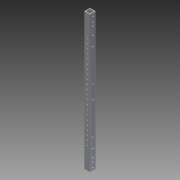
# Autodesk Inventor part: Chassis V1.500 Part1
Saved by Autodesk Inventor 2013 (Build 170138000, 138)
## iProperties
Created: 2013-01-05
Part Number: Chassis V1.500 Part1
Material: Aluminum 6061
Document SubType Name: Modeling
Designer: Moses
Density: 2.71 g/cm^3
Mass: 446.253 g
Surface Area: 1087.72 cm^2
Volume: 164.669 cm^3
Author: Moses
Autodesk Inventor part; units mm, degrees
ref_plane "YZ Plane" through (0, 0, 0) normal (1, 0, 0) x (0, 1, 0)
ref_plane "XZ Plane" through (0, 0, 0) normal (0, 1, 0) x (-1, 0, 0)
ref_plane "XY Plane" through (0, 0, 0) normal (0, 0, 1) x (1, 0, 0)
sketch "Sketch1" plane through (0, 0, 0) normal (0, 1, 0) x (-1, 0, 0)
  line L0 (0, 25.4) -> (25.4, 25.4)
  line L1 (25.4, 25.4) -> (25.4, 0)
  line L2 (25.4, 0) -> (0, 0)
  line L3 (0, 0) -> (0, 25.4)
  line L4 (22.225, 22.225) -> (3.175, 22.225)
  line L5 (3.175, 22.225) -> (3.175, 3.175)
  line L6 (3.175, 3.175) -> (22.225, 3.175)
  line L7 (22.225, 3.175) -> (22.225, 22.225)
  dimension "d0" = 25.4
  dimension "d1" = 25.4
  dimension "d2" = 3.175
  constraints: 16 end point, 4 parallel, 2 perpendicular, 1 coincident, 1 horizontal, 3 other
  measures "d0" distance of L1.end L2.end
  measures "d1" distance of L0.end L1.end
  measures "d2" distance between parallel lines of L0 L4
extrude "Extrusion1" add sketch "Sketch1" along normal blind 609.6
sketch "Sketch2" plane through (-25.4, 0, 25.4) normal (0, 0, 1) x (1, 0, 0)
  circle A0 centre (12.7, 491.5841) radius 3.302 projected
  circle A1 centre (12.7, 452.2611) radius 3.302 projected
  circle A2 centre (12.7, 412.9381) radius 3.302 projected
  circle A3 centre (12.7, 373.6152) radius 3.302 projected
  circle A4 centre (12.7, 334.2922) radius 3.302 projected
  circle A5 centre (12.7, 294.9693) radius 3.302 projected
  circle A6 centre (12.7, 255.6463) radius 3.302 projected
  circle A7 centre (12.7, 216.3233) radius 3.302 projected
  circle A8 centre (12.7, 177.0004) radius 3.302 projected
  circle A9 centre (12.7, 137.6774) radius 3.302 projected
  circle A10 centre (12.7, 98.3544) radius 3.302 projected
  circle A11 centre (12.7, 118.0159) radius 3.302 projected
  circle A12 centre (12.7, 157.3389) radius 3.302 projected
  circle A13 centre (12.7, 196.6619) radius 3.302 projected
  circle A14 centre (12.7, 235.9848) radius 3.302 projected
  circle A15 centre (12.7, 275.3078) radius 3.302 projected
  circle A16 centre (12.7, 314.6307) radius 3.302 projected
  circle A17 centre (12.7, 353.9537) radius 3.302 projected
  circle A18 centre (12.7, 393.2767) radius 3.302 projected
  circle A19 centre (12.7, 432.5996) radius 3.302 projected
  circle A20 centre (12.7, 471.9226) radius 3.302 projected
  circle A21 centre (12.7, 511.2456) radius 3.302 projected
  line L0 (0, 25.4) -> (25.4, 25.4) projected
  line L1 (0, 25.4) -> (0, 584.2) projected
  line L2 (25.4, 584.2) -> (0, 584.2) projected
  line L3 (25.4, 25.4) -> (25.4, 584.2) projected
extrude "Extrusion2" cut sketch "Sketch2" against normal through all contours A0 | A1 | A2 | A3 | A4 | A5 | A6 | A7 | A8 | A9 | A10 | A11 | A12 | A13 | A14 | A15 | A16 | A17 | A18 | A19 | A20 | A21
sketch "Sketch3" plane through (-25.4, 0, 0) normal (-1, 0, 0) x (0, 0, 1)
  line L0 (25.4, 0) -> (25.4, 609.6) projected
  line L1 (0, 0) -> (0, 609.6) projected
  line L2 (0, 511.2456) -> (25.4, 511.2456) construction
  line L3 (0, 373.6152) -> (25.4, 373.6152) construction
  line L4 (0, 235.9848) -> (25.4, 235.9848) construction
  line L5 (0, 98.3544) -> (25.4, 98.3544) construction
  line L6 (12.7, 523.9456) -> (12.7, 479.4956) construction
  line L7 (12.7, 403.7777) -> (12.7, 343.4527) construction
  line L8 (12.7, 258.2098) -> (12.7, 213.7598) construction
  line L9 (12.7, 130.1044) -> (12.7, 85.6544) construction
  circle A0 centre (12.7, 523.9456) radius 3.302
  circle A1 centre (12.7, 479.4956) radius 3.302
  circle A2 centre (12.7, 403.7777) radius 3.302
  circle A3 centre (12.7, 343.4527) radius 3.302
  circle A4 centre (12.7, 258.2098) radius 3.302
  circle A5 centre (12.7, 213.7598) radius 3.302
  circle A6 centre (12.7, 130.1044) radius 3.302
  circle A7 centre (12.7, 85.6544) radius 3.302
  line L10 (0, 304.8) -> (25.4, 304.8) construction
  line L11 (12.7, 334.9625) -> (12.7, 274.6375) construction
  circle A8 centre (12.7, 334.9625) radius 3.302
  circle A9 centre (12.7, 274.6375) radius 3.302
  line L12 (0, 609.6) -> (25.4, 609.6) projected
  line L13 (0, 107.8794) -> (25.4, 107.8794) construction
  line L14 (25.4, 0) -> (0, 0) projected
  circle A10 centre (12.7, 596.9) radius 3.302 projected
  circle A11 centre (12.7, 574.675) radius 3.302 projected
  circle A12 centre (12.7, 558.8) radius 3.302 projected
  line L15 (0, 501.7206) -> (25.4, 501.7206) construction
  circle A13 centre (12.7, 12.7) radius 3.302 projected
  circle A14 centre (12.7, 34.925) radius 3.302 projected
  circle A15 centre (12.7, 50.8) radius 3.302 projected
  line L16 (22.225, 507.9436) -> (22.225, 514.5476) projected
  line L17 (22.225, 95.0524) -> (22.225, 101.6564) projected
  line L18 (22.225, 232.6828) -> (22.225, 239.2868) projected
  line L19 (22.225, 370.3132) -> (22.225, 376.9172) projected
  point P0 (12.7, 235.9848)
  point P1 (12.7, 373.6152)
  point P2 (12.7, 304.8)
  point P3 (12.7, 107.8794)
  point P4 (12.7, 501.7206)
  point P5 (22.225, 511.2456)
  point P6 (22.225, 373.6152)
  point P7 (22.225, 235.9848)
  point P8 (22.225, 98.3544)
  dimension "d7" = 44.45
  dimension "d8" = 60.325
  dimension "d9" = 44.45
  dimension "d10" = 44.45
  dimension "d11" = 6.604
  dimension "d12" = 6.604
  dimension "d13" = 6.604
  dimension "d14" = 6.604
  dimension "d15" = 6.604
  dimension "d16" = 6.604
  dimension "d17" = 6.604
  dimension "d18" = 6.604
  dimension "d21" = 60.325
  dimension "d22" = 6.604
  dimension "d23" = 6.604
  dimension "d27" = 9.525
  dimension "d28" = 9.525
  constraints: 24 end point, 14 midpoint, 10 centre point, 10 coincident, 4 point on line, 3 collinear, 3 horizontal, 3 parallel, 2 perpendicular, 16 other
  measures "d7" distance of L6.start L6.end
  measures "d8" distance of L7.start L7.end
  measures "d9" distance of L8.start L8.end
  measures "d10" distance of L9.start L9.end
  measures "d11" diameter of A0
  measures "d12" diameter of A1
  measures "d13" diameter of A2
  measures "d14" diameter of A3
  measures "d15" diameter of A4
  measures "d16" diameter of A5
  measures "d17" diameter of A6
  measures "d18" diameter of A7
  measures "d21" distance of L11.start L11.end
  measures "d22" diameter of A8
  measures "d23" diameter of A9
  measures "d27" distance between parallel lines of L5 L13
  measures "d28" distance between parallel lines of L15 L2
extrude "Extrusion3" cut sketch "Sketch3" against normal blind 25.4 contours A0 | A1 | A6 | A7 | A8 | A9 | A10 | A11 | A12 | A13 | A14 | A15
equation "\"d9\" = d7"
equation "\"d10\" = d7"
equation "\"d12\" = d11"
equation "\"d13\" = d11"
equation "\"d14\" = d11"
equation "\"d15\" = d11"
equation "\"d16\" = d11"
equation "\"d17\" = d11"
equation "\"d18\" = d11"
equation "\"d21\" = d8"
equation "\"d22\" = d11"
equation "\"d23\" = d11"
equation "\"d27\" = d28"
body "Solid1"
